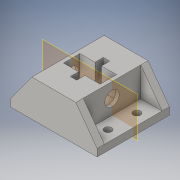
# Autodesk Inventor part: Ythruster
Saved by Autodesk Inventor 2016 (Build 200138000, 138)
## iProperties
Created: 2016-04-20
Part Number: Ythruster
Material: Generic
Document SubType Name: Modeling
Designer: Scott
Density: 1 g/cm^3
Appearance: Default
Author: Scott
Autodesk Inventor part; units mm, degrees
ref_plane "YZ Plane" through (0, 0, 0) normal (1, 0, 0) x (0, 1, 0)
ref_plane "XZ Plane" through (0, 0, 0) normal (0, 1, 0) x (-1, 0, 0)
ref_plane "XY Plane" through (0, 0, 0) normal (0, 0, 1) x (1, 0, 0)
sketch "Sketch1" plane through (0, 0, 0) normal (0, 1, 0) x (-1, 0, 0)
  line L0 (0, 0) -> (60, 0)
  line L1 (60, 0) -> (60, -40)
  line L2 (60, -40) -> (0, -40)
  line L3 (0, -40) -> (0, 0)
  line L4 (0, -20) -> (60, -20)
  line L5 (0, 0) -> (0, -20)
  line L6 (0, -10) -> (7.5, -10)
  line L7 (0, -10) -> (7.5, -10) construction
  circle A0 centre (7.5, -10) radius 2.5
  line L8 (60, -10) -> (52.5, -10)
  circle A1 centre (52.5, -10) radius 2.5
  circle A2 centre (7.5, -30) radius 2.5
  circle A3 centre (52.5, -30) radius 2.5
  dimension "d0" = 60
  dimension "d1" = 40
  dimension "d2" = 7.5
  dimension "d3" = 0
  dimension "d4" = 5
  dimension "d5" = 7.5
  dimension "d6" = 5
  constraints: 18 end point, 4 centre point, 3 horizontal, 3 midpoint, 3 perpendicular, 2 coincident, 2 parallel, 2 symmetric about line, 1 collinear, 1 point on line, 2 other
  measures "d0" distance of L1.end L2.end
  measures "d1" distance of L0.end L1.end
  measures "d2" distance of L6.start L6.end
  measures "d3" distance between parallel lines of L6 L7
  measures "d4" diameter of A0
  measures "d5" distance of L8.start L8.end
  measures "d6" diameter of A1
extrude "Extrusion1" add sketch "Sketch1" along normal blind 5.08
ref_plane "Work Plane1" through (-30, 0, -40) normal (-1, 0, 0) x (0, 0, 1)
sketch "Sketch2" plane through (-30, 0, -40) normal (-1, 0, 0) x (0, 0, 1)
  line L0 (40, 0) -> (0, 0) projected
  line L1 (0, 0) -> (0, 5.08) projected
  line L2 (40, 5.08) -> (0, 5.08) projected
  line L3 (40, 0) -> (40, 5.08) projected
  line L4 (0, 0) -> (40, 0) projected
  line L5 (20, 0) -> (20, 25.4)
  line L6 (20, 25.4) -> (20, 15.24)
  line L7 (7.3, 5.08) -> (32.7, 5.08)
  line L8 (32.7, 5.08) -> (32.7, 25.4)
  line L9 (32.7, 25.4) -> (7.3, 25.4)
  line L10 (7.3, 25.4) -> (7.3, 5.08)
  line L11 (7.3, 5.08) -> (32.7, 25.4) construction
  line L12 (32.7, 5.08) -> (7.3, 25.4) construction
  dimension "d9" = 25.4
  dimension "d10" = 10.16
  dimension "d11" = 25.4
  constraints: 16 end point, 3 midpoint, 2 parallel, 1 horizontal, 1 perpendicular, 1 point on line, 1 vertical
  measures "d9" distance of L5.start L5.end
  measures "d10" distance of L5.end L6.end
  measures "d11" distance of L9.end L8.end
extrude "Extrusion2" add sketch "Sketch2" along normal mid plane 30.48 contours L5 L9 L8 L2 | L2 L10 L9 L5
sketch "Sketch3" plane through (-45.24, 25.4, -32.7) normal (0, 1, 0) x (1, 0, 0)
  line L0 (30.48, 0) -> (0, 0) projected
  line L1 (0, -25.4) -> (0, 0) projected
  line L2 (30.48, -25.4) -> (0, -25.4) projected
  line L3 (30.48, 0) -> (30.48, -25.4) projected
  line L4 (17.4625, -1.27) -> (13.0175, -1.27)
  line L5 (13.0175, -1.27) -> (13.0175, -24.13)
  line L6 (13.0175, -24.13) -> (17.4625, -24.13)
  line L7 (17.4625, -24.13) -> (17.4625, -1.27)
  line L8 (17.4625, -1.27) -> (13.0175, -24.13) construction
  line L9 (13.0175, -1.27) -> (17.4625, -24.13) construction
  line L10 (27.94, -6.985) -> (2.54, -6.985)
  line L11 (2.54, -6.985) -> (2.54, -18.415)
  line L12 (2.54, -18.415) -> (27.94, -18.415)
  line L13 (27.94, -18.415) -> (27.94, -6.985)
  line L14 (27.94, -6.985) -> (2.54, -18.415) construction
  line L15 (2.54, -6.985) -> (27.94, -18.415) construction
  point P0 (45.24, -32.7)
  point P1 (15.24, -12.7)
  point P2 (15.24, -12.7)
  dimension "d14" = 4.445
  dimension "d15" = 22.86
  dimension "d16" = 25.4
  dimension "d17" = 11.43
  constraints: 24 end point, 5 midpoint, 4 parallel, 2 horizontal, 2 perpendicular
  measures "d14" distance of L6.end L5.end
  measures "d15" distance of L5.end L4.end
  measures "d16" distance of L12.end L11.end
  measures "d17" distance of L11.end L10.end
extrude "Extrusion3" cut sketch "Sketch3" against normal blind 20.32 contours L7 L10 L5 L4 | L10 L13 L12 L7 | L7 L12 L5 L10 | L5 L12 L11 L10 | L7 L6 L5 L12
fillet "Fillet1" radius 5.08 4 edges at (-37.4613, 5.08, -25.715) (-37.4613, 5.08, -14.285) (-22.5388, 5.08, -14.285) (-22.5388, 5.08, -25.715)
fillet "Fillet2" radius 10.16 2 edges at (-30, 5.08, -31.43) (-30, 5.08, -8.57)
sketch "Sketch4" plane through (-42.7, 25.4, -14.285) normal (1, 0, 0) x (0, 0, -1)
  arc A0 (0, -15.24) -> (5.08, -20.32) centre (5.08, -15.24) ccw projected
  line L0 (5.08, -20.32) -> (6.35, -20.32) projected
  arc A1 (6.35, -20.32) -> (11.43, -15.24) centre (6.35, -15.24) ccw projected
  line L1 (11.43, 0) -> (11.43, -15.24) projected
  line L2 (0, 0) -> (11.43, 0) projected
  line L3 (0, 0) -> (0, -15.24) projected
  line L4 (5.715, 0) -> (5.715, -10.16)
  line L5 (5.715, 0) -> (15.875, 0) construction
  circle A2 centre (5.715, -10.16) radius 5
  point P0 (-14.285, -25.4)
  dimension "d22" = 10.16
  dimension "d23" = 90
  dimension "d24" = 10
  constraints: 4 end point, 1 centre point, 1 coincident, 1 horizontal, 1 midpoint, 1 perpendicular, 1 vertical
  measures "d22" distance of L4.start L4.end
  measures "d23" angle of L4 L5
  measures "d24" diameter of A2
extrude "Extrusion4" cut sketch "Sketch4" along normal mid plane 117.1575 contours A2
sketch "Sketch5" plane through (0, 0, -40) normal (0, 0, -1) x (-1, 0, 0)
  line L0 (10, 0) -> (10, 5.08) projected
  line L1 (0, 0) -> (60, 0) projected
  line L2 (60, 0) -> (60, 5.08) projected
  line L3 (0, 5.08) -> (60, 5.08) projected
  line L4 (0, 0) -> (0, 5.08) projected
  line L5 (45.24, 5.08) -> (14.76, 5.08) projected
  line L6 (45.24, 25.4) -> (45.24, 5.08) projected
  line L7 (14.76, 25.4) -> (45.24, 25.4) projected
  line L8 (14.76, 5.08) -> (14.76, 25.4) projected
  line L9 (14.76, 25.4) -> (0, 5.08)
  line L10 (45.24, 5.08) -> (45.24, 25.4) projected
  line L11 (45.24, 25.4) -> (60, 5.08)
  constraints: 4 end point
extrude "Extrusion5" add sketch "Sketch5" along normal blind 5.08
sketch "Sketch6" plane through (-14.76, 5.08, -32.7) normal (0, 0, -1) x (-1, 0, 0)
  line L0 (13.0175, 0) -> (2.54, 0) projected
  line L1 (30.48, 0) -> (0, 0) projected
  line L2 (30.48, 20.32) -> (30.48, 0) projected
  line L3 (0, 20.32) -> (30.48, 20.32) projected
  line L4 (0, 0) -> (0, 20.32) projected
  point P0 (-14.76, -5.08)
extrude "Extrusion6" add sketch "Sketch6" along normal up to surface (7.3 mm away)
ref_plane "Work Plane2" through (-27.7775, 25.4, -20) normal (0, 0, 1) x (1, 0, 0)
mirror "Mirror1" about plane through (-27.7775, 25.4, -20) normal (0, 0, 1) of "Extrusion5", "Extrusion6"
body "Solid1"
